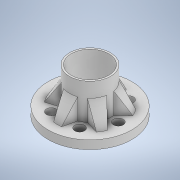
# Autodesk Inventor part: Connector_ring
Saved by Autodesk Inventor 2022 (Build 260153000, 153)
## iProperties
Created: 2021-12-14
Part Number: Connector_ring
Material: Generic
Document SubType Name: Modeling
Designer: Emazuddin Alif
Density: 1 g/cm^3
Appearance: Default
Author: Emazuddin Alif
Autodesk Inventor part; units mm, degrees
ref_plane "YZ Plane" through (0, 0, 0) normal (1, 0, 0) x (0, 1, 0)
ref_plane "XZ Plane" through (0, 0, 0) normal (0, 1, 0) x (-1, 0, 0)
ref_plane "XY Plane" through (0, 0, 0) normal (0, 0, 1) x (1, 0, 0)
sketch "Sketch1" plane through (0, 0, 0) normal (0, 0, 1) x (1, 0, 0)
  line L0 (0, 52.767) -> (0, -45.7542)
  line L1 (-13.335, 25.4) -> (-13.335, 0)
  line L2 (-10.5093, 0) -> (-10.5092, -6.0071)
  line L3 (-13.335, 0) -> (-10.5093, 0)
  line L4 (-13.335, 25.4) -> (-14.605, 25.4)
  line L5 (-14.605, 25.4) -> (-14.605, 14.903)
  line L6 (-10.5092, -6.0071) -> (-29.7815, -6.0071)
  line L7 (-29.7815, -6.0071) -> (-29.7815, 0)
  line L8 (-29.7815, 0) -> (-23.2093, 0)
  line L9 (-23.2093, 0) -> (-14.605, 14.903)
  point P0 (0, 0)
  dimension "d0" = 25.4
  dimension "d1" = 26.67
  dimension "d2" = 6.0071
  dimension "d3" = 21.0185
  dimension "d4" = 1.27
  dimension "d5" = 19.2722
  dimension "d6" = 6.5723
  dimension "d7" = 30
  constraints: 20 end point, 5 vertical, 2 horizontal, 2 perpendicular, 1 point on line
  measures "d0" distance of L1.start L1.end
  measures "d1" diameter of L1 L0
  measures "d2" distance of L2.start L2.end
  measures "d3" diameter of L2 L0
  measures "d4" distance of L1.start L4.end
  measures "d5" distance of L2.end L6.end
  measures "d6" distance of L7.end L8.end
  measures "d7" angle of L5 L9
revolve "Revolution1" add sketch "Sketch1" angle 360 about axis through (0, 52.767, 0) along (0, -1, 0)
sketch "Sketch2" plane through (0, -6.0071, 0) normal (0, -1, 0) x (1, 0, 0)
  circle A0 centre (0, 0) radius 10.5093
  circle A1 centre (0, 0) radius 10.5092 projected
  circle A2 centre (0, 0) radius 29.7815
  circle A3 centre (0, 0) radius 20.1454
  circle A4 centre (0, 0) radius 29.7815 projected
  line L0 (29.7815, 0) -> (20.1454, 0)
  line L1 (-10.5093, 0) -> (-20.1454, 0)
  circle A5 centre (20.1454, 0) radius 3.4925
  circle A6 centre (10.0727, 17.4464) radius 3.4925
  circle A7 centre (-10.0727, 17.4464) radius 3.4925
  circle A8 centre (-20.1454, 0) radius 3.4925
  circle A9 centre (-10.0727, -17.4464) radius 3.4925
  circle A10 centre (10.0727, -17.4464) radius 3.4925
  point P0 (0, 0)
  dimension "d10" = 6.985
  dimension "d13" = 360
  constraints: 9 centre point, 4 coincident, 4 end point, 2 horizontal alignment, 2 point on circle, 2 point on line, 1 collinear, 1 horizontal, 15 other
  measures "d10" diameter of A5
extrude "Extrusion1" cut sketch "Sketch2" against normal through all contours A8 A3 L1 | L1 A3 A8 | A3 A8 | A7 A3 | A3 A7 | A9 A3 | A3 A9 | A6 A3 | A3 A6 | A10 A3 | A3 A10 | A5 L0 A3 | A3 A5 | A3 L0 A5
sketch "Sketch3" plane through (0, 0, 0) normal (0, 1, 0) x (1, 0, 0)
  circle A0 centre (0, 0) radius 29.7815 projected
  arc A1 (26.4165, -13.7516) -> (26.4165, 13.7516) centre (0, 0) ccw
  line L0 (14.3942, 2.4722) -> (26.4165, 13.7516)
  line L1 (14.3942, -2.4722) -> (26.4165, -13.7516)
  circle A2 centre (0, 0) radius 14.605 projected
  arc A3 (14.3942, -2.4722) -> (14.3942, 2.4722) centre (0, 0) ccw
  arc A4 (25.1175, 16.0016) -> (1.2991, 29.7532) centre (0, 0) ccw
  line L2 (5.0561, 13.7019) -> (1.2991, 29.7532)
  line L3 (9.3381, 11.2297) -> (25.1175, 16.0016)
  arc A5 (9.3381, 11.2297) -> (5.0561, 13.7019) centre (0, 0) ccw
  arc A6 (-1.2991, 29.7532) -> (-25.1175, 16.0016) centre (0, 0) ccw
  line L4 (-9.3381, 11.2297) -> (-25.1175, 16.0016)
  line L5 (-5.0561, 13.7019) -> (-1.2991, 29.7532)
  arc A7 (-5.0561, 13.7019) -> (-9.3381, 11.2297) centre (0, 0) ccw
  arc A8 (-26.4165, 13.7516) -> (-26.4165, -13.7516) centre (0, 0) ccw
  line L6 (-14.3942, -2.4722) -> (-26.4165, -13.7516)
  line L7 (-14.3942, 2.4722) -> (-26.4165, 13.7516)
  arc A9 (-14.3942, 2.4722) -> (-14.3942, -2.4722) centre (0, 0) ccw
  arc A10 (-25.1175, -16.0016) -> (-1.2991, -29.7532) centre (0, 0) ccw
  line L8 (-5.0561, -13.7019) -> (-1.2991, -29.7532)
  line L9 (-9.3381, -11.2297) -> (-25.1175, -16.0016)
  arc A11 (-9.3381, -11.2297) -> (-5.0561, -13.7019) centre (0, 0) ccw
  arc A12 (1.2991, -29.7532) -> (25.1175, -16.0016) centre (0, 0) ccw
  line L10 (9.3381, -11.2297) -> (25.1175, -16.0016)
  line L11 (5.0561, -13.7019) -> (1.2991, -29.7532)
  arc A13 (5.0561, -13.7019) -> (9.3381, -11.2297) centre (0, 0) ccw
  line L12 (-2.8655, 0) -> (7.3025, 0)
  point P0 (23.1395, -1.798)
  point P1 (23.1395, 1.798)
  point P2 (19.5399, 3.4396)
  point P3 (19.5399, -3.4396)
  point P4 (13.1269, 19.1404)
  point P5 (10.0126, 20.9384)
  point P6 (-10.0126, 20.9384)
  point P7 (-13.1269, 19.1404)
  point P8 (-23.1395, 1.798)
  point P9 (-23.1395, -1.798)
  point P10 (-13.1269, -19.1404)
  point P11 (-10.0126, -20.9384)
  point P12 (10.0126, -20.9384)
  point P13 (13.1269, -19.1404)
  point P14 (-5.0561, 13.7019)
  point P15 (-1.2991, 29.7532)
  point P16 (-25.1175, 16.0016)
  point P17 (-9.3381, 11.2297)
  point P18 (-14.3942, 2.4722)
  point P19 (-26.4165, 13.7516)
  point P20 (-26.4165, -13.7516)
  point P21 (-14.3942, -2.4722)
  point P22 (-9.3381, -11.2297)
  point P23 (-25.1175, -16.0016)
  point P24 (-1.2991, -29.7532)
  point P25 (-5.0561, -13.7019)
  point P26 (5.0561, -13.7019)
  point P27 (1.2991, -29.7532)
  point P28 (25.1175, -16.0016)
  point P29 (9.3381, -11.2297)
  point P30 (9.3381, 11.2297)
  point P31 (1.2991, 29.7532)
  point P32 (5.0561, 13.7019)
  dimension "d21" = 360
  dimension "d23" = 55
  constraints: 28 point on circle, 26 end point, 12 centre point, 2 coincident, 1 horizontal, 75 other
extrude "Extrusion2" cut sketch "Sketch3" along normal blind 25.4 contours A0 L1 A2 L0 | L3 A2 L2 A0 | A0 L11 A2 L10 | L5 A2 L4 A0 | A0 L9 A2 L8 | L7 A2 L6 A0
body "Solid1"
